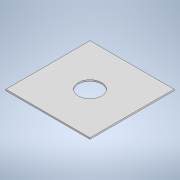
# Autodesk Inventor part: Tapa
Saved by Autodesk Inventor 2020.1 (Build 241239000, 239)
## iProperties
Created: 2020-03-26
Part Number: Tapa
Material: Generic
Document SubType Name: Modeling
Designer: Daniel
Density: 1 g/cm^3
Appearance: Default
Author: Daniel
Autodesk Inventor part; units mm, degrees
ref_plane "YZ Plane" through (0, 0, 0) normal (1, 0, 0) x (0, 1, 0)
ref_plane "XZ Plane" through (0, 0, 0) normal (0, 1, 0) x (-1, 0, 0)
ref_plane "XY Plane" through (0, 0, 0) normal (0, 0, 1) x (1, 0, 0)
sketch "Sketch1" plane through (0, 0, 0) normal (0, 1, 0) x (-1, 0, 0)
  line L0 (-87, 87) -> (87, 87) construction
  line L1 (87, 87) -> (87, -87) construction
  line L2 (87, -87) -> (-87, -87) construction
  line L3 (-87, -87) -> (-87, 87) construction
  line L4 (-87, 87) -> (87, -87) construction
  line L5 (87, 87) -> (-87, -87) construction
  line L6 (-90, 90) -> (90, 90)
  line L7 (90, 90) -> (90, -90)
  line L8 (90, -90) -> (-90, -90)
  line L9 (-90, -90) -> (-90, 90)
  line L10 (-90, 90) -> (90, -90) construction
  line L11 (90, 90) -> (-90, -90) construction
  point P0 (0, 0)
  dimension "d0" = 174
  dimension "d1" = 174
  dimension "d2" = 3
  constraints: 24 end point, 4 midpoint, 4 parallel, 2 horizontal, 2 perpendicular, 1 point on line
  measures "d0" distance of L1.end L2.end
  measures "d1" distance of L0.end L1.end
  measures "d2" distance between parallel lines of L2 L8
extrude "Extrusion1" add sketch "Sketch1" along normal blind 3
sketch "Sketch2" plane through (0, 3, 0) normal (0, 1, 0) x (1, 0, 0)
  circle A0 centre (0, 0) radius 25
  dimension "d5" = 50
  constraints: 1 centre point, 1 coincident
  measures "d5" diameter of A0
extrude "Extrusion2" cut sketch "Sketch2" against normal through all
body "Solid1"
